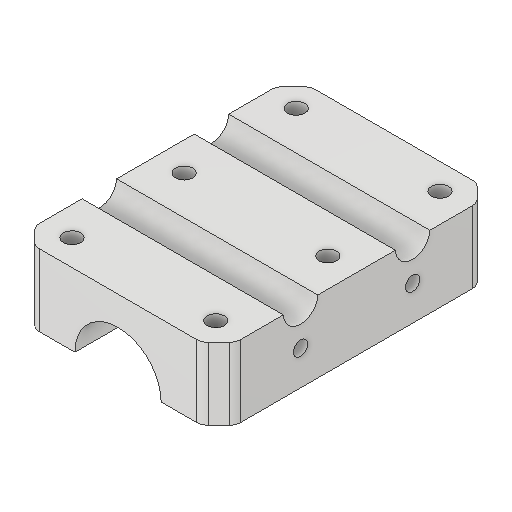
# Autodesk Inventor part: 3DP_PLA_X_end_top_half
Saved by Autodesk Inventor 2026.1 (Build 301233000, 233)
## iProperties
Created: 2018-07-03
Part Number: 3DP_PLA_X_end_top_half
Material: ABS Plastic
Document SubType Name: Modeling
Designer: Andrzej
Density: 1.06 g/cm^3
Appearance: Smooth - White
Author: Andrzej
Autodesk Inventor part; units mm, degrees
ref_plane "YZ Plane" through (0, 0, 0) normal (1, 0, 0) x (0, 1, 0)
ref_plane "XZ Plane" through (0, 0, 0) normal (0, 1, 0) x (-1, 0, 0)
ref_plane "XY Plane" through (0, 0, 0) normal (0, 0, 1) x (1, 0, 0)
sketch "Sketch1" plane through (0, 0, 0) normal (0, 0, 1) x (1, 0, 0)
  circle A0 centre (0, 0) radius 7.5
  line L0 (-17.5, 0) -> (-7.5, 0)
  line L1 (7.5, 0) -> (17.5, 0)
  line L2 (-17.5, 0) -> (-17.5, 12.5)
  line L3 (-17.5, 12.5) -> (17.5, 12.5)
  line L4 (17.5, 12.5) -> (17.5, 0)
  dimension "d5" = 15
  dimension "d6" = 0
  dimension "d8" = 0
  dimension "d11" = 10
  dimension "d13" = 10
  dimension "d19" = 12.5
  dimension "d76" = 35
  constraints: 10 end point, 3 horizontal, 2 point on circle, 1 centre point, 1 perpendicular, 1 vertical, 1 other
  measures "d5" diameter of A0
  measures "d6" distance from line of A0.centre L0
  measures "d8" distance from line of A0.centre L1
  measures "d11" distance of L0.start L0.end
  measures "d13" distance of L1.start L1.end
  measures "d19" distance from line of L3 A0.centre
  measures "d76" distance of L2.end L3.end
extrude "Extrusion1" add sketch "Sketch1" along normal blind 48 contours A0 L0 L2 L3 L4 L1
sketch "Sketch3" plane through (7.5, 0, 0) normal (0, -1, 0) x (1, 0, 0)
  line L0 (10, 0) -> (10, 48) projected
  line L1 (0, 48) -> (10, 48) projected
  line L2 (0, 0) -> (0, 48) projected
  line L3 (0, 0) -> (10, 0) projected
  line L4 (-25, 0) -> (-15, 0) projected
  line L5 (-15, 0) -> (-15, 48) projected
  line L6 (-25, 48) -> (-15, 48) projected
  line L7 (-25, 0) -> (-25, 48) projected
  point P0 (-7.5, 0)
  point P1 (5, 4.5)
  point P2 (5, 24)
  point P3 (5, 43.5)
  point P4 (-20, 43.5)
  point P5 (-20, 4.5)
  point P6 (-20, 24)
  dimension "d31" = 48
  dimension "d35" = 5
  dimension "d44" = 4.5
  dimension "d45" = 4.5
  dimension "d46" = 24
  dimension "d47" = 5
  dimension "d48" = 10
  dimension "d49" = 10
  constraints: 4 vertical alignment, 3 horizontal alignment
  measures "d31" distance between parallel lines of L3 L1
  measures "d35" distance from line of L7 point (-20, 4.5)
  measures "d44" distance from line of L4 point (-20, 4.5)
  measures "d45" distance from line of L6 point (-20, 43.5)
  measures "d46" distance from line of L4 point (-20, 24)
  measures "d47" horizontal distance of L0 point (5, 4.5)
  measures "d48" distance of L6.start L5.end
  measures "d49" distance of L1.start L0.end
hole "Hole1" at (12.5, 0, 4.5) at (12.5, 0, 24) at (12.5, 0, 43.5) at (-12.5, 0, 43.5) at (-12.5, 0, 4.5) at (-12.5, 0, 24) direction (0, 1, 0) diameter 3 end through all
sketch "Sketch4" plane through (17.5, 0, 0) normal (1, 0, 0) x (0, 0, -1)
  line L0 (0, 0) -> (0, 12.5) projected
  line L1 (0, 12.5) -> (-48, 12.5) projected
  line L2 (-48, 0) -> (-48, 12.5) projected
  line L3 (0, 0) -> (-48, 0) projected
  line L4 (0, 12.5) -> (-48, 12.5) projected
  circle A0 centre (-33.75, 12.6) radius 3
  circle A1 centre (-14.25, 12.6) radius 3
  dimension "d54" = 6
  dimension "d55" = 6
  dimension "d56" = 14.25
  dimension "d57" = 14.25
  dimension "d58" = 0.1
  dimension "d59" = 0.1
  constraints: 2 centre point
  measures "d54" diameter of A0
  measures "d55" diameter of A1
  measures "d56" distance from line of L2 A0.centre
  measures "d57" distance from line of L0 A1.centre
  measures "d58" distance from line of L1 A0.centre
  measures "d59" distance from line of L1 A1.centre
extrude "Extrusion3" cut sketch "Sketch4" against normal through all contours A1 L1 | L1 A1 | A0 L1 | L1 A0
chamfer "Chamfer1" distance 3 angle 45 4 edges at (17.5, 6.25, 48) (-17.5, 6.25, 48) (17.5, 6.25, 0) (-17.5, 6.25, 0)
fillet "Fillet2" radius 2 8 edges at (17.5, 6.25, 45) (14.5, 6.25, 48) (-14.5, 6.25, 48) (-17.5, 6.25, 45) (-17.5, 6.25, 3) (-14.5, 6.25, 0) (14.5, 6.25, 0) (17.5, 6.25, 3)
sketch "Sketch5" plane through (17.5, 12.5, 30.7517) normal (1, 0, 0) x (0, 0, -1)
  line L0 (-17.2483, 0) -> (-17.2483, -12.5) projected
  line L1 (30.7517, -12.5) -> (30.7517, 0) projected
  line L2 (26.9232, -12.5) -> (-13.4199, -12.5) projected
  point P0 (-2.9983, -6.5)
  point P1 (16.5017, -6.5)
  dimension "d66" = 6
  dimension "d67" = 14.25
  dimension "d68" = 14.25
  constraints: 1 horizontal alignment
  measures "d66" distance from line of L2 point (-2.998, -6.5)
  measures "d67" distance from line of L0 point (-2.998, -6.5)
  measures "d68" distance from line of L1 point (16.502, -6.5)
hole "Hole2" at (17.5, 6, 33.75) at (17.5, 6, 14.25) direction (-1, 0, 0) diameter 2.5 depth 10 tip angle 118
equation "\"d13\" = d11"
equation "\"d35\" = 0.5 * d48"
equation "\"d45\" = d44"
equation "\"d46\" = 0.5 * d31"
equation "\"d47\" = d35"
equation "\"d57\" = d56"
equation "\"d68\" = d67"
body "Solid1"
